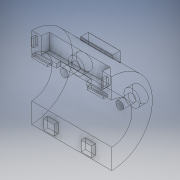
# Autodesk Inventor part: Slider Mount_A
Saved by Autodesk Inventor 2018 (Build 220112000, 112)
## iProperties
Created: 2018-01-05
Part Number: Slider Mount_A
Material: Generic
Document SubType Name: Modeling
Designer: njcfu
Density: 1 g/cm^3
Appearance: Default
Author: njcfu
Autodesk Inventor part; units mm, degrees
ref_plane "YZ Plane" through (0, 0, 0) normal (1, 0, 0) x (0, 1, 0)
ref_plane "XZ Plane" through (0, 0, 0) normal (0, 1, 0) x (-1, 0, 0)
sketch "Sketch1" plane through (0, 0, 0) normal (1, 0, 0) x (0, 1, 0)
  arc A0 (-25.4, 0) -> (25.4, 0) centre (0, 0) ccw
  arc A1 (-12.7, 0) -> (12.7, 0) centre (0, 0) ccw
  line L0 (25.4, 0) -> (12.7, 0)
  line L1 (-12.7, 0) -> (-25.4, 0)
  line L2 (0, 5.08) -> (0, -30.48) projected
  dimension "d0" = 25.4
  dimension "d1" = 12.7
  dimension "d5" = 12.7
  dimension "d6" = 12.7
  dimension "d7" = 270
  dimension "d8" = 90
  constraints: 5 point on circle, 4 end point, 2 centre point, 2 coincident
  measures "d0" radius of A0
  measures "d1" radius of A1
  measures "d5" distance of L1.start L1.end
  measures "d6" distance of L0.start L0.end
  measures "d8" angle of L2 L1
extrude "Extrusion1" add sketch "Sketch1" along normal mid plane 49.9999
ref_plane "Work Plane2" through (0, 0, -25.4) normal (0, 0, 1) x (1, 0, 0)
sketch "Sketch10" plane through (0, 0, -25.4) normal (0, 0, 1) x (1, 0, 0)
  circle A0 centre (17.38, 0) radius 5.08
  circle A1 centre (-17.38, 0) radius 5.08
  line L0 (25, -25.4) -> (25, 25.4) projected
  line L1 (-25, 25.4) -> (-25, 25.4) projected
  line L2 (25, -25.4) -> (-25, -25.4) projected
  point P0 (0, 0)
  dimension "d62" = 7.62
  dimension "d63" = 7.62
  dimension "d66" = 10.16
  dimension "d67" = 10.16
  dimension "d86" = 0
  dimension "d87" = 0
  constraints: 2 centre point
  measures "d62" distance from line of L0 A0.centre
  measures "d63" distance from line of L1 A1.centre
  measures "d66" diameter of A0
  measures "d67" diameter of A1
  measures "d86" vertical distance of point (0, 0) A0.centre
  measures "d87" vertical distance of point (0, 0) A1.centre
extrude "Extrusion7" cut sketch "Sketch10" along normal blind 5.08
sketch "Sketch12" plane through (0, 0, 0) normal (0, 0, 1) x (1, 0, 0)
  circle A0 centre (-17.38, 0) radius 2.413
  circle A1 centre (17.38, 0) radius 2.413
  line L0 (-25, 25.4) -> (25, 25.4) projected
  line L1 (-25, 25.4) -> (-25, 25.4) projected
  line L2 (25, 25.4) -> (25, 25.4) projected
  point P0 (0, 0)
  dimension "d78" = 4.826
  dimension "d79" = 4.826
  dimension "d82" = 7.62
  dimension "d83" = 7.62
  dimension "d88" = 0
  dimension "d89" = 0
  constraints: 2 centre point
  measures "d78" diameter of A0
  measures "d79" diameter of A1
  measures "d82" distance from line of L1 A0.centre
  measures "d83" distance from line of L2 A1.centre
  measures "d88" vertical distance of point (0, 0) A1.centre
  measures "d89" vertical distance of point (0, 0) A0.centre
extrude "Extrusion9" cut sketch "Sketch12" along normal mid plane 50.8
sketch "Sketch13" plane through (-25, 12.7, 0) normal (0, 0, 1) x (1, 0, 0)
  line L0 (2.54, 0.635) -> (12.7, 0.635)
  line L1 (12.7, 0.635) -> (12.7, 1.905)
  line L2 (12.7, 1.905) -> (2.54, 1.905)
  line L3 (2.54, 1.905) -> (2.54, 0.635)
  line L4 (37.2999, 1.905) -> (47.4599, 1.905)
  line L5 (47.4599, 1.905) -> (47.4599, 0.635)
  line L6 (47.4599, 0.635) -> (37.2999, 0.635)
  line L7 (37.2999, 0.635) -> (37.2999, 1.905)
  line L8 (49.9999, 12.7) -> (49.9999, 0) projected
  line L9 (0, 0) -> (0, 12.7) projected
  line L10 (49.9999, 0) -> (0, 0) projected
  point P0 (25, -12.7)
  dimension "d90" = 10.16
  dimension "d92" = 10.16
  dimension "d93" = 2.54
  dimension "d105" = 0.635
  dimension "d106" = 0.635
  dimension "d107" = 2.54
  dimension "d108" = 1.27
  constraints: 16 end point, 4 parallel, 2 horizontal, 2 perpendicular, 1 point on line
  measures "d90" distance of L1.end L2.end
  measures "d92" distance of L4.start L4.end
  measures "d93" distance between parallel lines of L3 L9
  measures "d105" distance between parallel lines of L10 L0
  measures "d106" distance between parallel lines of L10 L6
  measures "d107" distance between parallel lines of L8 L5
  measures "d108" distance of L4.end L5.end
extrude "Extrusion10" add sketch "Sketch13" along normal blind 2.54
ref_plane "Work Plane6" through (0, 15.24, 0) normal (0, 1, 0) x (1, 0, 0)
sketch "Sketch16" plane through (0, 15.24, 0) normal (0, 1, 0) x (1, 0, 0)
  line L0 (-9.525, -2.54) -> (9.525, -2.54)
  line L1 (9.525, -2.54) -> (9.525, 2.54)
  line L2 (9.525, 2.54) -> (-9.525, 2.54)
  line L3 (-9.525, 2.54) -> (-9.525, -2.54)
  line L4 (-9.525, -2.54) -> (9.525, 2.54) construction
  line L5 (9.525, -2.54) -> (-9.525, 2.54) construction
  point P0 (0, 0)
  dimension "d109" = 19.05
  dimension "d110" = 5.08
  constraints: 12 end point, 2 midpoint, 2 parallel, 1 horizontal, 1 perpendicular
  measures "d109" distance of L0.start L0.end
  measures "d110" distance of L0.end L1.end
extrude "Extrusion13" cut sketch "Sketch16" against normal blind 25.4
sketch "Sketch18" plane through (-25, 12.7, 0) normal (0, 0, 1) x (1, 0, 0)
  line L0 (3.556, 6.35) -> (2.286, 6.35)
  line L1 (2.286, 6.35) -> (2.286, 11.43)
  line L2 (2.286, 11.43) -> (3.556, 11.43)
  line L3 (3.556, 11.43) -> (3.556, 6.35)
  line L4 (3.556, 6.35) -> (2.286, 11.43) construction
  line L5 (2.286, 6.35) -> (3.556, 11.43) construction
  line L6 (47.7139, 6.35) -> (46.4439, 6.35)
  line L7 (46.4439, 6.35) -> (46.4439, 11.43)
  line L8 (46.4439, 11.43) -> (47.7139, 11.43)
  line L9 (47.7139, 11.43) -> (47.7139, 6.35)
  line L10 (47.7139, 6.35) -> (46.4439, 11.43) construction
  line L11 (46.4439, 6.35) -> (47.7139, 11.43) construction
  line L12 (0, 0) -> (0, 12.7) projected
  line L13 (0, 12.7) -> (49.9999, 12.7) projected
  line L14 (49.9999, 12.7) -> (49.9999, 0) projected
  line L15 (0, 12.7) -> (49.9999, 12.7) projected
  point P0 (25, -12.7)
  point P1 (2.921, 8.89)
  point P2 (47.0789, 8.89)
  point P3 (5.95, 12.7)
  point P4 (44.05, 12.7)
  dimension "d133" = 1.27
  dimension "d134" = 5.08
  dimension "d135" = 1.27
  dimension "d136" = 5.08
  dimension "d137" = 2.286
  dimension "d138" = 1.27
  dimension "d139" = 2.286
  dimension "d140" = 1.27
  constraints: 24 end point, 4 midpoint, 4 parallel, 2 horizontal, 2 perpendicular
  measures "d133" distance of L0.start L0.end
  measures "d134" distance of L0.end L1.end
  measures "d135" distance of L6.start L6.end
  measures "d136" distance of L8.end L6.start
  measures "d137" distance between parallel lines of L12 L1
  measures "d138" distance between parallel lines of L13 L2
  measures "d139" distance between parallel lines of L14 L9
  measures "d140" distance between parallel lines of L15 L8
extrude "Extrusion15" add sketch "Sketch18" along normal blind 2.54
sketch "Sketch19" plane through (-25, -25.4, 0) normal (0, 0, 1) x (1, 0, 0)
  line L0 (10.16, 3.175) -> (16.51, 3.175)
  line L1 (16.51, 3.175) -> (16.51, 9.525)
  line L2 (16.51, 9.525) -> (10.16, 9.525)
  line L3 (10.16, 9.525) -> (10.16, 3.175)
  line L4 (10.16, 3.175) -> (16.51, 9.525) construction
  line L5 (16.51, 3.175) -> (10.16, 9.525) construction
  line L6 (33.4899, 3.175) -> (39.8399, 3.175)
  line L7 (39.8399, 3.175) -> (39.8399, 9.525)
  line L8 (39.8399, 9.525) -> (33.4899, 9.525)
  line L9 (33.4899, 9.525) -> (33.4899, 3.175)
  line L10 (33.4899, 3.175) -> (39.8399, 9.525) construction
  line L11 (39.8399, 3.175) -> (33.4899, 9.525) construction
  line L12 (49.9999, 0) -> (0, 0) projected
  line L13 (0, 0) -> (0, 12.7) projected
  line L14 (49.9999, 12.7) -> (49.9999, 0) projected
  point P0 (25, 25.4)
  point P1 (13.335, 6.35)
  point P2 (36.6649, 6.35)
  dimension "d143" = 6.35
  dimension "d144" = 6.35
  dimension "d145" = 3.175
  dimension "d146" = 10.16
  dimension "d147" = 10.16
  dimension "d148" = 6.35
  dimension "d149" = 6.35
  dimension "d150" = 3.175
  constraints: 24 end point, 4 midpoint, 4 parallel, 2 horizontal, 2 perpendicular
  measures "d143" distance of L2.end L0.start
  measures "d144" distance of L0.start L0.end
  measures "d145" distance between parallel lines of L12 L0
  measures "d146" distance between parallel lines of L13 L3
  measures "d147" distance between parallel lines of L14 L7
  measures "d148" distance of L6.start L6.end
  measures "d149" distance of L6.end L7.end
  measures "d150" distance between parallel lines of L12 L6
extrude "Extrusion16" add sketch "Sketch19" along normal blind 2.54
ref_plane "Work Plane5" through (0, 25.4, 0) normal (0, 1, 0) x (-1, 0, 0)
sketch "Sketch20" plane through (0, 25.4, 0) normal (0, 1, 0) x (-1, 0, 0)
  line L0 (19.05, 5.08) -> (-19.05, 5.08)
  line L1 (-19.05, 5.08) -> (-19.05, -5.08)
  line L2 (-19.05, -5.08) -> (19.05, -5.08)
  line L3 (19.05, -5.08) -> (19.05, 5.08)
  line L4 (19.05, 5.08) -> (-19.05, -5.08) construction
  line L5 (-19.05, 5.08) -> (19.05, -5.08) construction
  point P0 (0, 0)
  dimension "d153" = 38.1
  dimension "d154" = 10.16
  constraints: 12 end point, 2 midpoint, 2 parallel, 1 horizontal, 1 perpendicular
  measures "d153" distance of L0.start L0.end
  measures "d154" distance of L0.end L1.end
extrude "Extrusion17" cut sketch "Sketch20" against normal blind 10.16
sketch "Sketch21" plane through (0, 0, 0) normal (1, 0, 0) x (0, 1, 0)
  line L0 (-12.7, 0) -> (-25.4, 0) projected
  arc A0 (-25.4, 0) -> (25.4, 0) centre (0, 0) ccw projected
  line L1 (0, 0) -> (17.9605, -17.9605)
  line L2 (25.4, 0) -> (12.7, 0) projected
  line L3 (14.1505, -15.4205) -> (21.7705, -15.4205)
  line L4 (21.7705, -15.4205) -> (21.7705, -20.5005)
  line L5 (21.7705, -20.5005) -> (14.1505, -20.5005)
  line L6 (14.1505, -20.5005) -> (14.1505, -15.4205)
  dimension "d172" = 45
  dimension "d173" = 5.08
  dimension "d174" = 2.54
  dimension "d175" = 7.62
  dimension "d176" = 3.81
  constraints: 10 end point, 2 parallel, 1 horizontal, 1 perpendicular, 1 point on circle
  measures "d172" angle of L2 L1
  measures "d173" distance of L5.end L3.start
  measures "d174" distance from line of L1.end L3
  measures "d175" distance of L4.end L5.end
  measures "d176" distance from line of L1.end L4
extrude "Extrusion18" add sketch "Sketch21" along normal mid plane 20
fillet "Fillet5" radius 0.254 2 edges at (0, 21.7705, -20.5005) (0, 21.7705, -15.4205)
body "Solid1"
